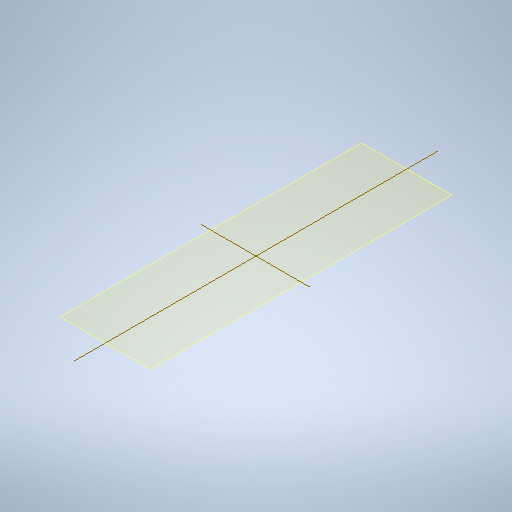
# Autodesk Inventor part: LoopPlane1
Saved by Autodesk Inventor 2025 (Build 290162010, 162A)
## iProperties
Created: 2024-08-27
Part Number: LoopPlane1
Material: Generic
Document SubType Name: Modeling
Designer: User
Density: 1 g/cm^3
Appearance: Default
Author: User
Autodesk Inventor part; units mm, degrees
ref_plane "YZ Plane" through (0, 0, 0) normal (1, 0, 0) x (0, 1, 0)
ref_plane "XZ Plane" through (0, 0, 0) normal (0, 1, 0) x (-1, 0, 0)
ref_plane "XY Plane" through (0, 0, 0) normal (0, 0, 1) x (1, 0, 0)
sketch "Sketch1" plane through (0, 0, 0) normal (0, 1, 0) x (-1, 0, 0)
  line L0 (30, 100) -> (-30, 100)
  line L1 (-30, 100) -> (-30, -100)
  line L2 (-30, -100) -> (30, -100)
  line L3 (30, -100) -> (30, 100)
  line L4 (30, 100) -> (-30, -100) construction
  line L5 (-30, 100) -> (30, -100) construction
  point P0 (0, 0)
  dimension "d2" = 200
  dimension "d3" = 60
  constraints: 12 end point, 2 midpoint, 2 parallel, 1 horizontal, 1 perpendicular
  measures "d2" distance of L0.end L1.end
  measures "d3" distance of L1.end L2.end
extrude "Extrusion1" add sketch "Sketch1" along normal blind 0.1
body "Solid1"
